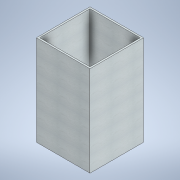
# Autodesk Inventor part: container
Saved by Autodesk Inventor 2021 (Build 250183000, 183)
## iProperties
Created: 2023-04-11
Part Number: container
Material: PC/ABS Plastic
Document SubType Name: Modeling
Designer: ASUS
Density: 0.357273 g/cm^3
Appearance: Wood - Painted White
Author: ASUS
Autodesk Inventor part; units mm, degrees
ref_plane "YZ Plane" through (0, 0, 0) normal (1, 0, 0) x (0, 1, 0)
ref_plane "XZ Plane" through (0, 0, 0) normal (0, 1, 0) x (-1, 0, 0)
ref_plane "XY Plane" through (0, 0, 0) normal (0, 0, 1) x (1, 0, 0)
sketch "Sketch1" plane through (0, 0, 0) normal (0, 1, 0) x (-1, 0, 0)
  line L0 (0, 0) -> (320, 0)
  line L1 (320, 0) -> (320, -320)
  line L2 (320, -320) -> (0, -320)
  line L3 (0, -320) -> (0, 0)
  dimension "d0" = 320
  dimension "d1" = 320
  constraints: 8 end point, 2 parallel, 1 horizontal, 1 perpendicular
  measures "d0" distance of L1.end L2.end
  measures "d1" distance between parallel lines of L2 L0
extrude "Extrusion1" add sketch "Sketch1" along normal blind 540
sketch "Sketch2" plane through (0, 540, 0) normal (0, 1, 0) x (1, 0, 0)
  line L0 (-310, 310) -> (-10, 310)
  line L1 (-10, 310) -> (-10, 10)
  line L2 (-10, 10) -> (-310, 10)
  line L3 (-310, 10) -> (-310, 310)
  line L4 (0, 320) -> (-320, 320) projected
  line L5 (-320, 0) -> (0, 0) projected
  line L6 (-320, 320) -> (-320, 0) projected
  line L7 (0, 0) -> (0, 320) projected
  dimension "d4" = 10
  dimension "d5" = 10
  dimension "d6" = 10
  dimension "d7" = 10
  constraints: 8 end point, 2 parallel, 1 horizontal, 1 perpendicular
  measures "d4" distance between parallel lines of L0 L4
  measures "d5" distance between parallel lines of L5 L2
  measures "d6" distance between parallel lines of L6 L3
  measures "d7" distance between parallel lines of L7 L1
extrude "Extrusion2" cut sketch "Sketch2" against normal blind 530 contours L0 L1 L2 L3
body "Solid1"
